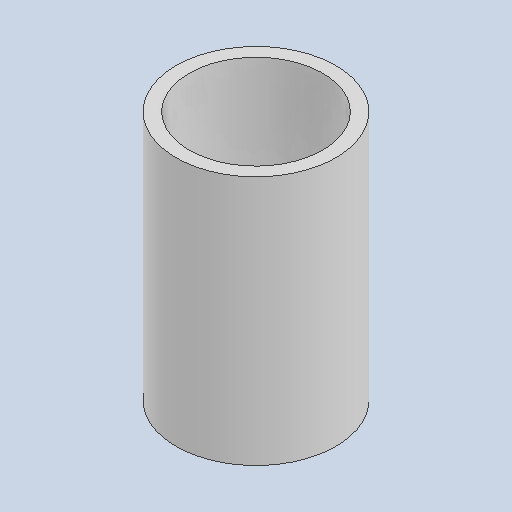
# Autodesk Inventor part: Thin_spacer_custom
Saved by Autodesk Inventor 2025.2 (Build 292293000, 293)
## iProperties
Created: 2024-12-08
Part Number: Thin_spacer_custom
Material: Generic
Document SubType Name: Modeling
Designer: Aditya Koduri
Density: 1 g/cm^3
Appearance: Default
Mass: 0.0487883 g
Surface Area: 2.45097 cm^2
Volume: 0.0487883 cm^3
Author: Aditya Koduri
Autodesk Inventor part; units mm, degrees
ref_plane "YZ Plane" through (0, 0, 0) normal (1, 0, 0) x (0, 1, 0)
ref_plane "XZ Plane" through (0, 0, 0) normal (0, 1, 0) x (-1, 0, 0)
ref_plane "XY Plane" through (0, 0, 0) normal (0, 0, 1) x (1, 0, 0)
sketch "Sketch1" plane through (0, 0, 0) normal (0, 1, 0) x (-1, 0, 0)
  circle A0 centre (0, 0) radius 2.54
  circle A1 centre (0, 0) radius 2.1209
  dimension "d0" = 5.08
  dimension "d1" = 4.2418
  constraints: 2 centre point, 2 coincident
  measures "d0" diameter of A0
  measures "d1" diameter of A1
extrude "Extrusion1" add sketch "Sketch1" along normal blind 7.9502
body "Solid1"
